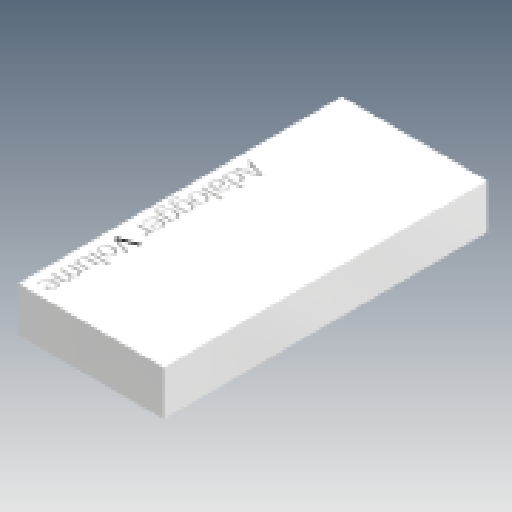
# Autodesk Inventor part: adalogger_mcu_volume
Saved by Autodesk Inventor 2025.4 (Build 294407020, 407B)
## iProperties
Created: 2026-09-16
Part Number: adalogger_mcu_volume
Material: Generic
Document SubType Name: Modeling
Designer: Aiden
Density: 1 g/cm^3
Appearance: Default
Author: Aiden
Autodesk Inventor part; units mm, degrees
ref_plane "YZ Plane" through (0, 0, 0) normal (1, 0, 0) x (0, 1, 0)
ref_plane "XZ Plane" through (0, 0, 0) normal (0, 1, 0) x (-1, 0, 0)
ref_plane "XY Plane" through (0, 0, 0) normal (0, 0, 1) x (1, 0, 0)
sketch "Sketch1" plane through (0, 0, 0) normal (0, 1, 0) x (-1, 0, 0)
  line L0 (0, 0) -> (-22.86, 0)
  line L1 (-22.86, 0) -> (-22.86, -50.8)
  line L2 (-22.86, -50.8) -> (0, -50.8)
  line L3 (0, -50.8) -> (0, 0)
  dimension "d0" = 50.8
  dimension "d1" = 22.86
  constraints: 8 end point, 2 parallel, 1 horizontal, 1 perpendicular
  measures "d0" distance of L0.end L1.end
  measures "d1" distance of L1.end L2.end
extrude "Extrusion1" add sketch "Sketch1" along normal blind 7
sketch "Sketch2" plane through (0, 7, 0) normal (0, 1, 0) x (1, 0, 0)
  line L0 (4.5317, 34.9694) -> (4.5317, 1.1456) construction
  line L1 (4.5317, 1.1456) -> (0.1494, 1.1456) construction
  line L2 (0.1494, 1.1456) -> (0.1494, 34.9694) construction
  line L3 (0.1494, 34.9694) -> (4.5317, 34.9694) construction
  line L4 (1.3478, 34.9892) -> (4.3958, 33.9616)
  line L5 (4.3958, 33.9616) -> (4.3958, 33.4627)
  line L6 (4.3958, 33.4627) -> (1.3478, 32.4352)
  line L7 (1.3478, 32.4352) -> (1.3478, 32.8625)
  line L8 (1.3478, 32.8625) -> (2.2, 33.1391)
  line L9 (2.2, 33.1391) -> (2.2, 34.3025)
  line L10 (2.2, 34.3025) -> (1.3478, 34.5791)
  line L11 (1.3478, 34.5791) -> (1.3478, 34.9892)
  line L12 (2.5458, 33.2503) -> (3.9809, 33.722)
  line L13 (3.9809, 33.722) -> (2.5458, 34.1913)
  line L14 (2.5458, 34.1913) -> (2.5458, 33.2503)
  line L15 (1.3478, 30.4172) -> (1.3478, 30.8025)
  line L16 (1.3478, 30.8025) -> (1.58, 30.8025)
  spline S0 degree 2 poles (1.58, 30.8025) (1.5059, 30.8914) (1.4071, 31.0223) (1.3651, 31.1112) knots 0 0 0 1 2 2 2
  spline S1 degree 2 poles (1.3651, 31.1112) (1.3256, 31.1927) (1.2836, 31.3681) (1.2836, 31.4842) knots 0 0 0 1 2 2 2
  spline S2 degree 2 poles (1.2836, 31.4842) (1.2836, 31.6719) (1.4392, 31.9881) (1.5899, 32.0992) knots 0 0 0 1 2 2 2
  spline S3 degree 2 poles (1.5899, 32.0992) (1.7406, 32.2104) (2.1852, 32.3339) (2.4742, 32.3339) knots 0 0 0 1 2 2 2
  spline S4 degree 2 poles (2.4742, 32.3339) (2.7755, 32.3339) (3.2152, 32.1783) (3.3807, 32.0424) knots 0 0 0 1 2 2 2
  spline S5 degree 2 poles (3.3807, 32.0424) (3.5289, 31.9165) (3.6993, 31.5632) (3.6993, 31.3681) knots 0 0 0 1 2 2 2
  spline S6 degree 2 poles (3.6993, 31.3681) (3.6993, 31.1977) (3.6227, 30.9433) (3.5437, 30.8025) knots 0 0 0 1 2 2 2
  line L17 (3.5437, 30.8025) -> (4.5317, 30.8025)
  line L18 (4.5317, 30.8025) -> (4.5317, 30.4172)
  line L19 (4.5317, 30.4172) -> (1.3478, 30.4172)
  line L20 (1.9036, 30.8025) -> (3.225, 30.8025)
  spline S7 degree 2 poles (3.225, 30.8025) (3.2942, 30.9457) (3.3461, 31.173) (3.3461, 31.3039) knots 0 0 0 1 2 2 2
  spline S8 degree 2 poles (3.3461, 31.3039) (3.3461, 31.6003) (2.9015, 31.9362) (2.4816, 31.9362) knots 0 0 0 1 2 2 2
  spline S9 degree 2 poles (2.4816, 31.9362) (2.0765, 31.9362) (1.6492, 31.6793) (1.6492, 31.3953) knots 0 0 0 1 2 2 2
  spline S10 degree 2 poles (1.6492, 31.3953) (1.6492, 31.2446) (1.7875, 30.9383) (1.9036, 30.8025) knots 0 0 0 1 2 2 2
  spline S11 degree 2 poles (1.5899, 28.5844) (1.5553, 28.6313) (1.4318, 28.7894) (1.3948, 28.8635) knots 0 0 0 1 2 2 2
  spline S12 degree 2 poles (1.3948, 28.8635) (1.3404, 28.9648) (1.2836, 29.155) (1.2836, 29.3279) knots 0 0 0 1 2 2 2
  spline S13 degree 2 poles (1.2836, 29.3279) (1.2836, 29.4687) (1.3898, 29.7231) (1.4862, 29.8194) knots 0 0 0 1 2 2 2
  spline S14 degree 2 poles (1.4862, 29.8194) (1.58, 29.9108) (1.8567, 30.022) (2.0098, 30.022) knots 0 0 0 1 2 2 2
  spline S15 degree 2 poles (2.0098, 30.022) (2.2469, 30.022) (2.5828, 29.8219) (2.6792, 29.6045) knots 0 0 0 1 2 2 2
  spline S16 degree 2 poles (2.6792, 29.6045) (2.7681, 29.4119) (2.8348, 28.8882) (2.8521, 28.5844) knots 0 0 0 1 2 2 2
  line L21 (2.8521, 28.5844) -> (2.9262, 28.5844)
  spline S17 degree 2 poles (2.9262, 28.5844) (3.0596, 28.5844) (3.225, 28.6659) (3.272, 28.74) knots 0 0 0 1 2 2 2
  spline S18 degree 2 poles (3.272, 28.74) (3.3189, 28.8141) (3.3486, 29.0265) (3.3486, 29.1402) knots 0 0 0 1 2 2 2
  spline S19 degree 2 poles (3.3486, 29.1402) (3.3486, 29.2735) (3.2695, 29.6342) (3.1929, 29.8145) knots 0 0 0 1 2 2 2
  line L22 (3.1929, 29.8145) -> (3.1929, 29.8367)
  line L23 (3.1929, 29.8367) -> (3.5857, 29.8367)
  spline S20 degree 2 poles (3.5857, 29.8367) (3.6153, 29.7305) (3.6894, 29.3328) (3.6894, 29.1377) knots 0 0 0 1 2 2 2
  spline S21 degree 2 poles (3.6894, 29.1377) (3.6894, 28.9006) (3.6153, 28.577) (3.519, 28.4486) knots 0 0 0 1 2 2 2
  spline S22 degree 2 poles (3.519, 28.4486) (3.4251, 28.3226) (3.1262, 28.1991) (2.9114, 28.1991) knots 0 0 0 1 2 2 2
  line L24 (2.9114, 28.1991) -> (1.3478, 28.1991)
  line L25 (1.3478, 28.1991) -> (1.3478, 28.5844)
  line L26 (1.3478, 28.5844) -> (1.5899, 28.5844)
  line L27 (1.911, 28.5844) -> (2.5458, 28.5844)
  spline S23 degree 2 poles (2.5458, 28.5844) (2.5334, 28.7227) (2.4915, 29.1402) (2.4519, 29.2711) knots 0 0 0 1 2 2 2
  spline S24 degree 2 poles (2.4519, 29.2711) (2.405, 29.4242) (2.2099, 29.6243) (2.037, 29.6243) knots 0 0 0 1 2 2 2
  spline S25 degree 2 poles (2.037, 29.6243) (1.8394, 29.6243) (1.6393, 29.402) (1.6393, 29.1896) knots 0 0 0 1 2 2 2
  spline S26 degree 2 poles (1.6393, 29.1896) (1.6393, 29.0092) (1.7949, 28.7128) (1.911, 28.5844) knots 0 0 0 1 2 2 2
  line L28 (1.3478, 27.2654) -> (1.3478, 27.6507)
  line L29 (1.3478, 27.6507) -> (4.5317, 27.6507)
  line L30 (4.5317, 27.6507) -> (4.5317, 27.2654)
  line L31 (4.5317, 27.2654) -> (1.3478, 27.2654)
  spline S27 degree 2 poles (2.4915, 24.8201) (1.9135, 24.8201) (1.2836, 25.3759) (1.2836, 25.8402) knots 0 0 0 1 2 2 2
  spline S28 degree 2 poles (1.2836, 25.8402) (1.2836, 26.3169) (1.9332, 26.8628) (2.4915, 26.8628) knots 0 0 0 1 2 2 2
  spline S29 degree 2 poles (2.4915, 26.8628) (3.0645, 26.8628) (3.6993, 26.2996) (3.6993, 25.8402) knots 0 0 0 1 2 2 2
  spline S30 degree 2 poles (3.6993, 25.8402) (3.6993, 25.3759) (3.067, 24.8201) (2.4915, 24.8201) knots 0 0 0 1 2 2 2
  spline S31 degree 2 poles (2.4915, 25.2178) (2.9361, 25.2178) (3.3683, 25.5413) (3.3683, 25.8402) knots 0 0 0 1 2 2 2
  spline S32 degree 2 poles (3.3683, 25.8402) (3.3683, 26.1391) (2.9361, 26.4651) (2.4915, 26.4651) knots 0 0 0 1 2 2 2
  spline S33 degree 2 poles (2.4915, 26.4651) (2.0592, 26.4651) (1.6146, 26.1391) (1.6146, 25.8402) knots 0 0 0 1 2 2 2
  spline S34 degree 2 poles (1.6146, 25.8402) (1.6146, 25.5438) (2.0518, 25.2178) (2.4915, 25.2178) knots 0 0 0 1 2 2 2
  spline S35 degree 2 poles (0.9823, 24.3434) (0.965, 24.3039) (0.9106, 24.1532) (0.8884, 24.0569) knots 0 0 0 1 2 2 2
  spline S36 degree 2 poles (0.8884, 24.0569) (0.8612, 23.9507) (0.8291, 23.7703) (0.8291, 23.6641) knots 0 0 0 1 2 2 2
  spline S37 degree 2 poles (0.8291, 23.6641) (0.8291, 23.4863) (0.923, 23.2393) (1.007, 23.1701) knots 0 0 0 1 2 2 2
  spline S38 degree 2 poles (1.007, 23.1701) (1.091, 23.1034) (1.3108, 23.0516) (1.4516, 23.0516) knots 0 0 0 1 2 2 2
  line L32 (1.4516, 23.0516) -> (1.6516, 23.0516)
  spline S39 degree 2 poles (1.6516, 23.0516) (1.5158, 23.2072) (1.3874, 23.506) (1.3874, 23.7308) knots 0 0 0 1 2 2 2
  spline S40 degree 2 poles (1.3874, 23.7308) (1.3874, 24.1211) (1.9678, 24.583) (2.5137, 24.583) knots 0 0 0 1 2 2 2
  spline S41 degree 2 poles (2.5137, 24.583) (2.7977, 24.583) (3.2374, 24.4224) (3.393, 24.289) knots 0 0 0 1 2 2 2
  spline S42 degree 2 poles (3.393, 24.289) (3.5387, 24.1606) (3.6993, 23.8074) (3.6993, 23.6197) knots 0 0 0 1 2 2 2
  spline S43 degree 2 poles (3.6993, 23.6197) (3.6993, 23.4418) (3.6153, 23.1825) (3.5387, 23.0516) knots 0 0 0 1 2 2 2
  line L33 (3.5387, 23.0516) -> (3.6351, 23.0293)
  line L34 (3.6351, 23.0293) -> (3.6351, 22.6662)
  line L35 (3.6351, 22.6662) -> (1.6097, 22.6662)
  spline S44 degree 2 poles (1.6097, 22.6662) (1.0267, 22.6662) (0.4833, 23.1726) (0.4833, 23.6938) knots 0 0 0 1 2 2 2
  spline S45 degree 2 poles (0.4833, 23.6938) (0.4833, 23.8617) (0.5377, 24.2125) (0.5821, 24.3631) knots 0 0 0 1 2 2 2
  line L36 (0.5821, 24.3631) -> (0.9823, 24.3631)
  line L37 (0.9823, 24.3631) -> (0.9823, 24.3434)
  line L38 (1.9678, 23.0516) -> (3.225, 23.0516)
  spline S46 degree 2 poles (3.225, 23.0516) (3.2942, 23.1948) (3.3535, 23.4369) (3.3535, 23.5579) knots 0 0 0 1 2 2 2
  spline S47 degree 2 poles (3.3535, 23.5579) (3.3535, 23.8494) (2.9237, 24.1853) (2.5211, 24.1853) knots 0 0 0 1 2 2 2
  spline S48 degree 2 poles (2.5211, 24.1853) (2.1407, 24.1853) (1.743, 23.9309) (1.743, 23.6444) knots 0 0 0 1 2 2 2
  spline S49 degree 2 poles (1.743, 23.6444) (1.743, 23.4937) (1.8616, 23.1775) (1.9678, 23.0516) knots 0 0 0 1 2 2 2
  spline S50 degree 2 poles (0.9823, 22.0265) (0.965, 21.987) (0.9106, 21.8363) (0.8884, 21.74) knots 0 0 0 1 2 2 2
  spline S51 degree 2 poles (0.8884, 21.74) (0.8612, 21.6338) (0.8291, 21.4535) (0.8291, 21.3473) knots 0 0 0 1 2 2 2
  spline S52 degree 2 poles (0.8291, 21.3473) (0.8291, 21.1694) (0.923, 20.9224) (1.007, 20.8533) knots 0 0 0 1 2 2 2
  spline S53 degree 2 poles (1.007, 20.8533) (1.091, 20.7866) (1.3108, 20.7347) (1.4516, 20.7347) knots 0 0 0 1 2 2 2
  line L39 (1.4516, 20.7347) -> (1.6516, 20.7347)
  spline S54 degree 2 poles (1.6516, 20.7347) (1.5158, 20.8903) (1.3874, 21.1892) (1.3874, 21.4139) knots 0 0 0 1 2 2 2
  spline S55 degree 2 poles (1.3874, 21.4139) (1.3874, 21.8042) (1.9678, 22.2661) (2.5137, 22.2661) knots 0 0 0 1 2 2 2
  spline S56 degree 2 poles (2.5137, 22.2661) (2.7977, 22.2661) (3.2374, 22.1055) (3.393, 21.9722) knots 0 0 0 1 2 2 2
  spline S57 degree 2 poles (3.393, 21.9722) (3.5387, 21.8437) (3.6993, 21.4905) (3.6993, 21.3028) knots 0 0 0 1 2 2 2
  spline S58 degree 2 poles (3.6993, 21.3028) (3.6993, 21.125) (3.6153, 20.8656) (3.5387, 20.7347) knots 0 0 0 1 2 2 2
  line L40 (3.5387, 20.7347) -> (3.6351, 20.7125)
  line L41 (3.6351, 20.7125) -> (3.6351, 20.3494)
  line L42 (3.6351, 20.3494) -> (1.6097, 20.3494)
  spline S59 degree 2 poles (1.6097, 20.3494) (1.0267, 20.3494) (0.4833, 20.8557) (0.4833, 21.3769) knots 0 0 0 1 2 2 2
  spline S60 degree 2 poles (0.4833, 21.3769) (0.4833, 21.5449) (0.5377, 21.8956) (0.5821, 22.0463) knots 0 0 0 1 2 2 2
  line L43 (0.5821, 22.0463) -> (0.9823, 22.0463)
  line L44 (0.9823, 22.0463) -> (0.9823, 22.0265)
  line L45 (1.9678, 20.7347) -> (3.225, 20.7347)
  spline S61 degree 2 poles (3.225, 20.7347) (3.2942, 20.878) (3.3535, 21.12) (3.3535, 21.241) knots 0 0 0 1 2 2 2
  spline S62 degree 2 poles (3.3535, 21.241) (3.3535, 21.5325) (2.9237, 21.8684) (2.5211, 21.8684) knots 0 0 0 1 2 2 2
  spline S63 degree 2 poles (2.5211, 21.8684) (2.1407, 21.8684) (1.743, 21.614) (1.743, 21.3275) knots 0 0 0 1 2 2 2
  spline S64 degree 2 poles (1.743, 21.3275) (1.743, 21.1768) (1.8616, 20.8607) (1.9678, 20.7347) knots 0 0 0 1 2 2 2
  spline S65 degree 2 poles (1.296, 18.7982) (1.296, 19.3465) (1.911, 19.9492) (2.4791, 19.9492) knots 0 0 0 1 2 2 2
  spline S66 degree 2 poles (2.4791, 19.9492) (3.0373, 19.9492) (3.6993, 19.3638) (3.6993, 18.8921) knots 0 0 0 1 2 2 2
  spline S67 degree 2 poles (3.6993, 18.8921) (3.6993, 18.6796) (3.5758, 18.3511) (3.4449, 18.2301) knots 0 0 0 1 2 2 2
  spline S68 degree 2 poles (3.4449, 18.2301) (3.314, 18.1066) (2.9361, 17.9757) (2.6619, 17.9757) knots 0 0 0 1 2 2 2
  line L46 (2.6619, 17.9757) -> (2.4519, 17.9757)
  line L47 (2.4519, 17.9757) -> (2.4519, 19.559)
  spline S69 degree 2 poles (2.4519, 19.559) (2.0543, 19.559) (1.6319, 19.1588) (1.6319, 18.8031) knots 0 0 0 1 2 2 2
  spline S70 degree 2 poles (1.6319, 18.8031) (1.6319, 18.6772) (1.6887, 18.4326) (1.7332, 18.3338) knots 0 0 0 1 2 2 2
  spline S71 degree 2 poles (1.7332, 18.3338) (1.7826, 18.2301) (1.869, 18.0868) (1.9085, 18.0399) knots 0 0 0 1 2 2 2
  line L48 (1.9085, 18.0399) -> (1.9085, 18.0177)
  line L49 (1.9085, 18.0177) -> (1.4886, 18.0177)
  spline S72 degree 2 poles (1.4886, 18.0177) (1.4615, 18.0844) (1.3824, 18.2869) (1.3602, 18.3659) knots 0 0 0 1 2 2 2
  spline S73 degree 2 poles (1.3602, 18.3659) (1.3281, 18.4771) (1.296, 18.6599) (1.296, 18.7982) knots 0 0 0 1 2 2 2
  spline S74 degree 2 poles (2.7459, 18.3511) (2.9015, 18.3561) (3.1287, 18.4203) (3.2053, 18.482) knots 0 0 0 1 2 2 2
  spline S75 degree 2 poles (3.2053, 18.482) (3.2917, 18.5487) (3.3831, 18.7587) (3.3831, 18.9143) knots 0 0 0 1 2 2 2
  spline S76 degree 2 poles (3.3831, 18.9143) (3.3831, 19.0674) (3.2917, 19.2823) (3.2028, 19.3712) knots 0 0 0 1 2 2 2
  spline S77 degree 2 poles (3.2028, 19.3712) (3.1114, 19.4577) (2.8916, 19.5466) (2.7459, 19.559) knots 0 0 0 1 2 2 2
  line L50 (2.7459, 19.559) -> (2.7459, 18.3511)
  line L51 (3.2226, 16.3726) -> (3.2226, 16.3924)
  spline S78 degree 2 poles (3.2226, 16.3924) (3.2349, 16.4369) (3.2399, 16.5332) (3.2399, 16.5999) knots 0 0 0 1 2 2 2
  spline S79 degree 2 poles (3.2399, 16.5999) (3.2399, 16.7555) (3.104, 17.0618) (2.9706, 17.2001) knots 0 0 0 1 2 2 2
  line L52 (2.9706, 17.2001) -> (1.3478, 17.2001)
  line L53 (1.3478, 17.2001) -> (1.3478, 17.5854)
  line L54 (1.3478, 17.5854) -> (3.6351, 17.5854)
  line L55 (3.6351, 17.5854) -> (3.6351, 17.2001)
  line L56 (3.6351, 17.2001) -> (3.2942, 17.2001)
  spline S80 degree 2 poles (3.2942, 17.2001) (3.4819, 16.9901) (3.6351, 16.6765) (3.6351, 16.5283) knots 0 0 0 1 2 2 2
  spline S81 degree 2 poles (3.6351, 16.5283) (3.6351, 16.469) (3.6301, 16.4097) (3.6227, 16.3726) knots 0 0 0 1 2 2 2
  line L57 (3.6227, 16.3726) -> (3.2226, 16.3726)
  line L58 (4.3958, 12.5244) -> (1.3478, 13.5741)
  line L59 (1.3478, 13.5741) -> (1.3478, 14.0113)
  line L60 (1.3478, 14.0113) -> (4.3958, 15.0611)
  line L61 (4.3958, 15.0611) -> (4.3958, 14.6263)
  line L62 (4.3958, 14.6263) -> (1.8641, 13.7816)
  line L63 (1.8641, 13.7816) -> (4.3958, 12.9368)
  line L64 (4.3958, 12.9368) -> (4.3958, 12.5244)
  spline S82 degree 2 poles (2.4915, 10.3829) (1.9135, 10.3829) (1.2836, 10.9386) (1.2836, 11.403) knots 0 0 0 1 2 2 2
  spline S83 degree 2 poles (1.2836, 11.403) (1.2836, 11.8797) (1.9332, 12.4256) (2.4915, 12.4256) knots 0 0 0 1 2 2 2
  spline S84 degree 2 poles (2.4915, 12.4256) (3.0645, 12.4256) (3.6993, 11.8624) (3.6993, 11.403) knots 0 0 0 1 2 2 2
  spline S85 degree 2 poles (3.6993, 11.403) (3.6993, 10.9386) (3.067, 10.3829) (2.4915, 10.3829) knots 0 0 0 1 2 2 2
  spline S86 degree 2 poles (2.4915, 10.7805) (2.9361, 10.7805) (3.3683, 11.1041) (3.3683, 11.403) knots 0 0 0 1 2 2 2
  spline S87 degree 2 poles (3.3683, 11.403) (3.3683, 11.7018) (2.9361, 12.0279) (2.4915, 12.0279) knots 0 0 0 1 2 2 2
  spline S88 degree 2 poles (2.4915, 12.0279) (2.0592, 12.0279) (1.6146, 11.7018) (1.6146, 11.403) knots 0 0 0 1 2 2 2
  spline S89 degree 2 poles (1.6146, 11.403) (1.6146, 11.1066) (2.0518, 10.7805) (2.4915, 10.7805) knots 0 0 0 1 2 2 2
  line L65 (1.3478, 9.5949) -> (1.3478, 9.9802)
  line L66 (1.3478, 9.9802) -> (4.5317, 9.9802)
  line L67 (4.5317, 9.9802) -> (4.5317, 9.5949)
  line L68 (4.5317, 9.5949) -> (1.3478, 9.5949)
  line L69 (1.3478, 7.2509) -> (1.3478, 7.6362)
  line L70 (1.3478, 7.6362) -> (1.5998, 7.6362)
  spline S90 degree 2 poles (1.5998, 7.6362) (1.4442, 7.814) (1.2836, 8.1327) (1.2836, 8.3303) knots 0 0 0 1 2 2 2
  spline S91 degree 2 poles (1.2836, 8.3303) (1.2836, 8.4785) (1.3824, 8.7428) (1.4886, 8.8391) knots 0 0 0 1 2 2 2
  spline S92 degree 2 poles (1.4886, 8.8391) (1.5948, 8.9379) (1.9184, 9.0466) (2.1506, 9.0466) knots 0 0 0 1 2 2 2
  line L71 (2.1506, 9.0466) -> (3.6351, 9.0466)
  line L72 (3.6351, 9.0466) -> (3.6351, 8.6613)
  line L73 (3.6351, 8.6613) -> (2.3309, 8.6613)
  spline S93 degree 2 poles (2.3309, 8.6613) (2.1481, 8.6613) (1.9085, 8.6341) (1.8196, 8.5872) knots 0 0 0 1 2 2 2
  spline S94 degree 2 poles (1.8196, 8.5872) (1.7307, 8.5402) (1.6492, 8.3797) (1.6492, 8.229) knots 0 0 0 1 2 2 2
  spline S95 degree 2 poles (1.6492, 8.229) (1.6492, 8.0882) (1.8097, 7.7696) (1.9258, 7.6362) knots 0 0 0 1 2 2 2
  line L74 (1.9258, 7.6362) -> (3.6351, 7.6362)
  line L75 (3.6351, 7.6362) -> (3.6351, 7.2509)
  line L76 (3.6351, 7.2509) -> (1.3478, 7.2509)
  line L77 (1.3478, 4.0991) -> (2.6718, 4.0991)
  spline S96 degree 2 poles (2.6718, 4.0991) (2.8298, 4.0991) (3.0991, 4.1238) (3.1732, 4.1634) knots 0 0 0 1 2 2 2
  spline S97 degree 2 poles (3.1732, 4.1634) (3.2547, 4.2029) (3.3337, 4.3535) (3.3337, 4.4845) knots 0 0 0 1 2 2 2
  spline S98 degree 2 poles (3.3337, 4.4845) (3.3337, 4.603) (3.188, 4.8747) (3.0497, 5.018) knots 0 0 0 1 2 2 2
  spline S99 degree 2 poles (3.0497, 5.018) (3.0151, 5.0155) (2.9188, 5.0106) (2.8545, 5.0106) knots 0 0 0 1 2 2 2
  line L78 (2.8545, 5.0106) -> (1.3478, 5.0106)
  line L79 (1.3478, 5.0106) -> (1.3478, 5.3959)
  line L80 (1.3478, 5.3959) -> (2.6718, 5.3959)
  spline S100 degree 2 poles (2.6718, 5.3959) (2.8298, 5.3959) (3.0991, 5.4206) (3.1732, 5.4601) knots 0 0 0 1 2 2 2
  spline S101 degree 2 poles (3.1732, 5.4601) (3.2547, 5.4996) (3.3337, 5.6503) (3.3337, 5.7812) knots 0 0 0 1 2 2 2
  spline S102 degree 2 poles (3.3337, 5.7812) (3.3337, 5.9047) (3.1781, 6.1789) (3.0571, 6.3073) knots 0 0 0 1 2 2 2
  line L81 (3.0571, 6.3073) -> (1.3478, 6.3073)
  line L82 (1.3478, 6.3073) -> (1.3478, 6.6926)
  line L83 (1.3478, 6.6926) -> (3.6351, 6.6926)
  line L84 (3.6351, 6.6926) -> (3.6351, 6.3073)
  line L85 (3.6351, 6.3073) -> (3.3831, 6.3073)
  spline S103 degree 2 poles (3.3831, 6.3073) (3.5338, 6.1567) (3.6993, 5.8603) (3.6993, 5.6824) knots 0 0 0 1 2 2 2
  spline S104 degree 2 poles (3.6993, 5.6824) (3.6993, 5.4799) (3.514, 5.1662) (3.3041, 5.0847) knots 0 0 0 1 2 2 2
  spline S105 degree 2 poles (3.3041, 5.0847) (3.4992, 4.9093) (3.6993, 4.5783) (3.6993, 4.3857) knots 0 0 0 1 2 2 2
  spline S106 degree 2 poles (3.6993, 4.3857) (3.6993, 4.2375) (3.6079, 3.9954) (3.5042, 3.9065) knots 0 0 0 1 2 2 2
  spline S107 degree 2 poles (3.5042, 3.9065) (3.4004, 3.8151) (3.0892, 3.7138) (2.8545, 3.7138) knots 0 0 0 1 2 2 2
  line L86 (2.8545, 3.7138) -> (1.3478, 3.7138)
  line L87 (1.3478, 3.7138) -> (1.3478, 4.0991)
  spline S108 degree 2 poles (1.296, 2.1799) (1.296, 2.7283) (1.911, 3.331) (2.4791, 3.331) knots 0 0 0 1 2 2 2
  spline S109 degree 2 poles (2.4791, 3.331) (3.0373, 3.331) (3.6993, 2.7456) (3.6993, 2.2738) knots 0 0 0 1 2 2 2
  spline S110 degree 2 poles (3.6993, 2.2738) (3.6993, 2.0614) (3.5758, 1.7329) (3.4449, 1.6118) knots 0 0 0 1 2 2 2
  spline S111 degree 2 poles (3.4449, 1.6118) (3.314, 1.4883) (2.9361, 1.3574) (2.6619, 1.3574) knots 0 0 0 1 2 2 2
  line L88 (2.6619, 1.3574) -> (2.4519, 1.3574)
  line L89 (2.4519, 1.3574) -> (2.4519, 2.9407)
  spline S112 degree 2 poles (2.4519, 2.9407) (2.0543, 2.9407) (1.6319, 2.5406) (1.6319, 2.1849) knots 0 0 0 1 2 2 2
  spline S113 degree 2 poles (1.6319, 2.1849) (1.6319, 2.0589) (1.6887, 1.8144) (1.7332, 1.7156) knots 0 0 0 1 2 2 2
  spline S114 degree 2 poles (1.7332, 1.7156) (1.7826, 1.6118) (1.869, 1.4686) (1.9085, 1.4216) knots 0 0 0 1 2 2 2
  line L90 (1.9085, 1.4216) -> (1.9085, 1.3994)
  line L91 (1.9085, 1.3994) -> (1.4886, 1.3994)
  spline S115 degree 2 poles (1.4886, 1.3994) (1.4615, 1.4661) (1.3824, 1.6686) (1.3602, 1.7477) knots 0 0 0 1 2 2 2
  spline S116 degree 2 poles (1.3602, 1.7477) (1.3281, 1.8588) (1.296, 2.0416) (1.296, 2.1799) knots 0 0 0 1 2 2 2
  spline S117 degree 2 poles (2.7459, 1.7329) (2.9015, 1.7378) (3.1287, 1.802) (3.2053, 1.8638) knots 0 0 0 1 2 2 2
  spline S118 degree 2 poles (3.2053, 1.8638) (3.2917, 1.9305) (3.3831, 2.1404) (3.3831, 2.296) knots 0 0 0 1 2 2 2
  spline S119 degree 2 poles (3.3831, 2.296) (3.3831, 2.4492) (3.2917, 2.6641) (3.2028, 2.753) knots 0 0 0 1 2 2 2
  spline S120 degree 2 poles (3.2028, 2.753) (3.1114, 2.8394) (2.8916, 2.9283) (2.7459, 2.9407) knots 0 0 0 1 2 2 2
  line L92 (2.7459, 2.9407) -> (2.7459, 1.7329)
  point P0 (0, 0)
  constraints: 2 other
emboss "Emboss1" sketch "Sketch2" operation cut depth 2 direction (0, -1, 0)
sketch "Sketch3" plane through (22.86, 0, -50.8) normal (0, 0, -1) x (-1, 0, 0)
  line L0 (8.1452, 2.0929) -> (14.7148, 2.0929)
  line L1 (14.7148, 2.0929) -> (14.7148, 4.9071)
  line L2 (14.7148, 4.9071) -> (8.1452, 4.9071)
  line L3 (8.1452, 4.9071) -> (8.1452, 2.0929)
  line L4 (0, 0) -> (0, 7) projected
  line L5 (0, 0) -> (22.86, 0) projected
  point P0 (8.1452, 3.5)
  point P1 (0, 3.5)
  point P2 (11.43, 2.0929)
  point P3 (11.43, 0)
  constraints: 8 end point, 4 midpoint, 2 parallel, 1 horizontal, 1 horizontal alignment, 1 perpendicular, 1 vertical alignment
extrude "Extrusion2" add sketch "Sketch3" along normal blind 1
body "Solid1"
